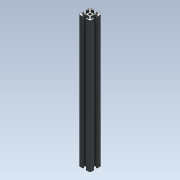
# Autodesk Inventor part: Profil_20x20_250
Saved by Autodesk Inventor 2022 (Build 260153000, 153)
## iProperties
Created: 2021-11-30
Part Number: Profil_20x20_250
Material: Generic
Document SubType Name: Modeling
Designer: Fabijan_Sven
Density: 1 g/cm^3
Appearance: Default
Author: Fabijan_Sven
Autodesk Inventor part; units mm, degrees
ref_plane "YZ Plane" through (0, 0, 0) normal (1, 0, 0) x (0, 1, 0)
ref_plane "XZ Plane" through (0, 0, 0) normal (0, 1, 0) x (-1, 0, 0)
ref_plane "XY Plane" through (0, 0, 0) normal (0, 0, 1) x (1, 0, 0)
sketch "Sketch1" plane through (0, 0, 0) normal (0, 1, 0) x (-1, 0, 0)
  line L0 (8, 10) -> (3, 10)
  line L1 (10, 3) -> (10, 8)
  line L2 (2.5, 9.5) -> (2.5, 8.2)
  line L3 (2.5, 8.2) -> (5.7198, 8.2)
  line L4 (6.0734, 7.3464) -> (3.2627, 4.5358)
  line L5 (1.8485, 3.95) -> (0, 3.95)
  line L6 (0, 3.95) -> (0, 2.15)
  line L7 (0, 2.15) -> (0, 2.15)
  line L8 (2.15, 0) -> (2.15, 0)
  line L9 (2.15, 0) -> (3.95, 0)
  line L10 (8.2, 5.7204) -> (8.2, 2.5)
  line L11 (8.2, 2.5) -> (9.5, 2.5)
  line L12 (0, 29.0836) -> (0, -4.1523) construction
  line L13 (3.95, 0) -> (3.95, 1.8491)
  line L14 (7.3464, 6.0739) -> (4.5358, 3.2633)
  arc A0 (10, 8) -> (8, 10) centre (8, 8) ccw
  arc A1 (8.2, 5.7204) -> (7.3464, 6.0739) centre (7.7, 5.7204) ccw
  arc A2 (6.0734, 7.3464) -> (5.7198, 8.2) centre (5.7198, 7.7) ccw
  arc A3 (4.5358, 3.2633) -> (3.95, 1.8491) centre (5.95, 1.8491) ccw
  arc A4 (1.8485, 3.95) -> (3.2627, 4.5358) centre (1.8485, 5.95) ccw
  arc A5 (2.15, 0) -> (0, 2.15) centre (0, 0) ccw
  arc A6 (3, 10) -> (2.5, 9.5) centre (3, 9.5) ccw
  arc A7 (9.5, 2.5) -> (10, 3) centre (9.5, 3) ccw
  line L15 (18.5462, 0) -> (-9.9601, 0) construction
  line L16 (-3, 10) -> (-8, 10)
  arc A8 (-2.5, 9.5) -> (-3, 10) centre (-3, 9.5) ccw
  line L17 (-2.5, 8.2) -> (-2.5, 9.5)
  line L18 (-5.7204, 8.2) -> (-2.5, 8.2)
  arc A9 (-5.7204, 8.2) -> (-6.0739, 7.3464) centre (-5.7204, 7.7) ccw
  line L19 (-6.0739, 7.3464) -> (-3.2633, 4.5358)
  arc A10 (-3.2633, 4.5358) -> (-1.8491, 3.95) centre (-1.8491, 5.95) ccw
  line L20 (0, 3.95) -> (-1.8491, 3.95)
  line L21 (0, 2.15) -> (0, 3.95)
  arc A11 (0, 2.15) -> (-2.15, 0) centre (0, 0) ccw
  line L22 (-3.95, 0) -> (-2.15, 0)
  line L23 (-3.95, 1.8485) -> (-3.95, 0)
  arc A12 (-3.95, 1.8485) -> (-4.5358, 3.2627) centre (-5.95, 1.8485) ccw
  line L24 (-7.3464, 6.0734) -> (-4.5358, 3.2627)
  arc A13 (-7.3464, 6.0734) -> (-8.2, 5.7198) centre (-7.7, 5.7198) ccw
  line L25 (-8.2, 2.5) -> (-8.2, 5.7198)
  line L26 (-9.5, 2.5) -> (-8.2, 2.5)
  arc A14 (-10, 3) -> (-9.5, 2.5) centre (-9.5, 3) ccw
  line L27 (-10, 8) -> (-10, 3)
  arc A15 (-8, 10) -> (-10, 8) centre (-8, 8) ccw
  line L28 (-10, -3) -> (-10, -8)
  arc A16 (-9.5, -2.5) -> (-10, -3) centre (-9.5, -3) ccw
  line L29 (-8.2, -2.5) -> (-9.5, -2.5)
  line L30 (-8.2, -5.7204) -> (-8.2, -2.5)
  arc A17 (-8.2, -5.7204) -> (-7.3464, -6.0739) centre (-7.7, -5.7204) ccw
  line L31 (-7.3464, -6.0739) -> (-4.5358, -3.2633)
  arc A18 (-4.5358, -3.2633) -> (-3.95, -1.8491) centre (-5.95, -1.8491) ccw
  line L32 (-3.95, 0) -> (-3.95, -1.8491)
  line L33 (-2.15, 0) -> (-3.95, 0)
  arc A19 (-2.15, 0) -> (0, -2.15) centre (0, 0) ccw
  line L34 (0, -3.95) -> (0, -2.15)
  line L35 (-1.8485, -3.95) -> (0, -3.95)
  arc A20 (-1.8485, -3.95) -> (-3.2627, -4.5358) centre (-1.8485, -5.95) ccw
  line L36 (-6.0734, -7.3464) -> (-3.2627, -4.5358)
  arc A21 (-6.0734, -7.3464) -> (-5.7198, -8.2) centre (-5.7198, -7.7) ccw
  line L37 (-2.5, -8.2) -> (-5.7198, -8.2)
  line L38 (-2.5, -9.5) -> (-2.5, -8.2)
  arc A22 (-3, -10) -> (-2.5, -9.5) centre (-3, -9.5) ccw
  line L39 (-8, -10) -> (-3, -10)
  arc A23 (-10, -8) -> (-8, -10) centre (-8, -8) ccw
  line L40 (3, -10) -> (8, -10)
  arc A24 (2.5, -9.5) -> (3, -10) centre (3, -9.5) ccw
  line L41 (2.5, -8.2) -> (2.5, -9.5)
  line L42 (5.7204, -8.2) -> (2.5, -8.2)
  arc A25 (5.7204, -8.2) -> (6.0739, -7.3464) centre (5.7204, -7.7) ccw
  line L43 (6.0739, -7.3464) -> (3.2633, -4.5358)
  arc A26 (3.2633, -4.5358) -> (1.8491, -3.95) centre (1.8491, -5.95) ccw
  line L44 (0, -3.95) -> (1.8491, -3.95)
  line L45 (0, -2.15) -> (0, -3.95)
  arc A27 (0, -2.15) -> (2.15, 0) centre (0, 0) ccw
  line L46 (3.95, 0) -> (2.15, 0)
  line L47 (3.95, -1.8485) -> (3.95, 0)
  arc A28 (3.95, -1.8485) -> (4.5358, -3.2627) centre (5.95, -1.8485) ccw
  line L48 (7.3464, -6.0734) -> (4.5358, -3.2627)
  arc A29 (7.3464, -6.0734) -> (8.2, -5.7198) centre (7.7, -5.7198) ccw
  line L49 (8.2, -2.5) -> (8.2, -5.7198)
  line L50 (9.5, -2.5) -> (8.2, -2.5)
  arc A30 (10, -3) -> (9.5, -2.5) centre (9.5, -3) ccw
  line L51 (10, -8) -> (10, -3)
  arc A31 (8, -10) -> (10, -8) centre (8, -8) ccw
  point P0 (0, 0)
  point P1 (3.95, 2.6775)
  point P2 (-2.6775, 3.95)
  point P3 (0, 0)
  point P4 (-3.95, -2.6775)
  point P5 (0, 0)
  point P6 (2.6775, -3.95)
  point P7 (0, 0)
  dimension "d1" = 2.5
  dimension "d2" = 2.5
  dimension "d3" = 1.8
  dimension "d4" = 1.8
  dimension "d5" = 45
  dimension "d6" = 2.15
  dimension "d7" = 2.15
  dimension "d8" = 1.8
  dimension "d11" = 10
  dimension "d12" = 10
  dimension "d14" = 1.8
  dimension "d15" = 1.8
  dimension "d16" = 2.6775
  dimension "d18" = 2
  dimension "d19" = 0.5
  dimension "d20" = 2
  dimension "d21" = 2.15
  dimension "d22" = 0.5
  dimension "d25" = 360
  constraints: 104 end point, 64 point on circle, 32 centre point, 16 point on line, 16 tangent, 5 perpendicular, 5 vertical, 3 equal radius, 3 parallel, 2 coincident, 2 horizontal, 207 other
  measures "d1" distance from line of point (0, 0) L2
  measures "d2" distance from line of point (0, 0) L11
  measures "d3" distance between parallel lines of L10 L1
  measures "d4" distance between parallel lines of L0 L3
  measures "d5" angle of L4 L12
  measures "d6" distance of point (0, 0) L6.end
  measures "d7" distance from line of point (0, 0) L8
  measures "d8" distance between parallel lines of L5 L7
  measures "d11" distance from line of point (0, 0) L0
  measures "d12" distance from line of point (0, 0) L1
  measures "d14" distance between parallel lines of L8 L13
  measures "d15" distance between parallel lines of L4 L14
  measures "d16" distance of L9.end point (3.95, 2.678)
  measures "d18" radius of A0
  measures "d19" radius of A1
  measures "d20" radius of A3
  measures "d21" radius of A5
  measures "d22" radius of A6
extrude "Profil_20x20" add sketch "Sketch1" along normal blind 230 contours A0 L1 A7 L11 L10 A1 L14 A3 L13 L9 A5 L6 L5 A4 L4 A2 L3 L2 A6 L0 | L6 A11 L22 L23 A12 L24 A13 L25 L26 A14 L27 A15 L16 A8 L17 L18 A9 L19 A10 L20 | L47 A28 L48 A29 L49 L50 A30 L51 A31 L40 A24 L41 L42 A25 L43 A26 L44 L34 A27 L9 | A19 L34 L35 A20 L36 A21 L37 L38 A22 L39 A23 L28 A16 L29 L30 A17 L31 A18 L32 L22
body "Solid1"
